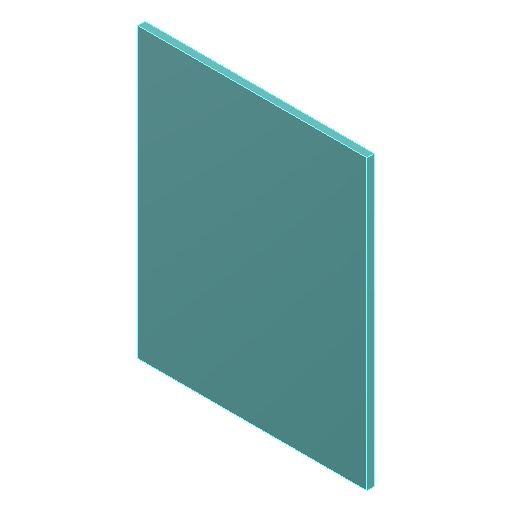
# Autodesk Inventor part: MH-ET_ESP32_D1_MINI
Saved by Autodesk Inventor 2022 (Build 260153000, 153)
## iProperties
Created: 2022-01-18
Part Number: MH-ET_ESP32_D1_MINI
Material: Generisch
Document SubType Name: Modeling
Designer: diederichbenedict
Density: 1 g/cm^3
Appearance: MH-ET_ESP32_D1_MINI, MH-ET_ESP32_D1_MINI
Author: diederichbenedict
Autodesk Inventor part; units mm, degrees
ref_plane "YZ Plane" through (0, 0, 0) normal (1, 0, 0) x (0, 1, 0)
ref_plane "XZ Plane" through (0, 0, 0) normal (0, 1, 0) x (-1, 0, 0)
ref_plane "XY Plane" through (0, 0, 0) normal (0, 0, 1) x (1, 0, 0)
sketch "MH-ET_ESP32_D1_MINI, MH-ET_ESP32_D1_MINI_3" plane through (0, 0, 0) normal (0, 0, 1) x (1, 0, 0)
  line L0 (-1.8135, 8.6135) -> (29.25, 8.6135)
  line L1 (29.25, 8.6135) -> (29.25, -30.5135)
  line L2 (29.25, -30.5135) -> (-1.8135, -30.5135)
  line L3 (-1.8135, -30.5135) -> (-1.8135, 8.6135)
  constraints: 8 end point
extrude "Extrusion1" add sketch "MH-ET_ESP32_D1_MINI, MH-ET_ESP32_D1_MINI_3" along normal blind 1
